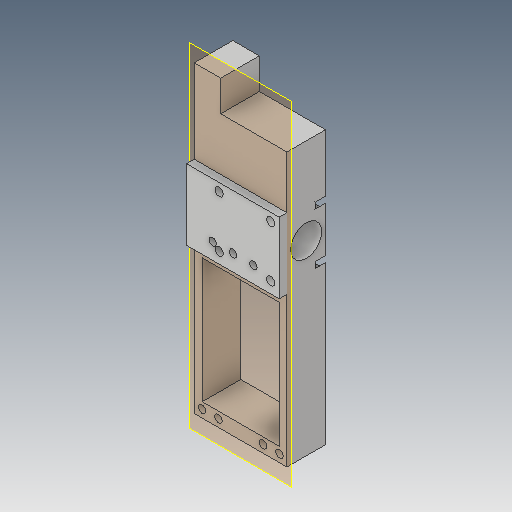
# Autodesk Inventor part: 01_Slide_camera_x_rail
Saved by Autodesk Inventor 2019.4 (Build 234330000, 330)
## iProperties
Created: 2021-01-10
Part Number: 01_Slide_camera_x_rail
Material: Generic
Document SubType Name: Modeling
Designer: diederichbenedict
Density: 1 g/cm^3
Appearance: Default
Author: diederichbenedict
Autodesk Inventor part; units mm, degrees
ref_plane "YZ Plane" through (0, 0, 0) normal (1, 0, 0) x (0, 1, 0)
ref_plane "XZ Plane" through (0, 0, 0) normal (0, 1, 0) x (-1, 0, 0)
ref_plane "Work Plane1" through (0, 0, 0) normal (0, 0, 1) x (1, 0, 0)
sketch "Sketch1" plane through (0, 0, 0) normal (0, 0, 1) x (1, 0, 0)
  line L0 (-14.0647, -9.1525) -> (-14.0647, 39.2801) projected
  line L1 (15.9353, 39.2801) -> (-14.0647, 39.2801) projected
  line L2 (15.9353, 39.2801) -> (15.9353, -9.1525) projected
  line L3 (15.9353, -9.1525) -> (-14.0647, -9.1525) projected
  circle A0 centre (13.8475, 49.7489) radius 1.45 projected
  circle A1 centre (-6.9768, 49.7489) radius 1.45 projected
  circle A2 centre (15.9823, -11.6603) radius 1.45 projected
  circle A3 centre (9.593, -11.6603) radius 1.45 projected
  circle A4 centre (-7.7223, -11.6603) radius 1.45 projected
  circle A5 centre (-14.1116, -11.6603) radius 1.45 projected
  circle A6 centre (8.8475, 49.7489) radius 1.45 projected
  circle A7 centre (-11.9768, 49.7489) radius 1.45 projected
  circle A8 centre (0.9375, 49.7489) radius 1.45 projected
  line L4 (-17.1585, 69.3865) -> (-2.1585, 69.3865) projected
  line L5 (-2.1585, 69.3865) -> (-2.1585, 62.7008) projected
  line L6 (-2.1585, 62.7008) -> (-2.1585, 59.9787) projected
  line L7 (-2.1585, 59.9787) -> (-2.1585, 53.293) projected
  line L8 (-2.1585, 53.293) -> (-17.1585, 53.293) projected
  line L9 (-17.1585, 53.293) -> (-17.1585, -14.6603) projected
  line L10 (-17.1585, -14.6603) -> (18.8415, -14.6603) projected
  line L11 (18.8415, -14.6603) -> (18.8415, 91.3397) projected
  line L12 (-6.8647, 91.3397) -> (18.8415, 91.3397) projected
  line L13 (-6.8647, 103.3397) -> (-6.8647, 91.3397) projected
  line L14 (-17.1585, 69.3865) -> (-17.1585, 103.3397) projected
  line L15 (-17.1585, 69.3865) -> (-17.1585, 53.293)
  line L16 (-17.1585, 103.3397) -> (-6.8647, 103.3397) projected
  point P0 (0, 0)
  constraints: 2 end point, 1 vertical
ref_plane "Work Plane2" through (-17.2444, -14.6603, -15) normal (0, 0, 1) x (1, 0, 0)
extrude "Extrusion1" add sketch "Sketch1" against normal up to surface (15 mm away) contours A0 | A7 | L14 L16 L13 L12 L11 L10 L9 L8 L7 L6 L5 L4 | L4 L5 L6 L7 L8 L15
sketch "Sketch2" plane through (-17.1585, -14.6603, 0) normal (-1, 0, 0) x (0, 0, 1)
  line L0 (-15, 0) -> (-15, 118) projected
  line L1 (0, 0) -> (-15, 0) projected
  line L2 (0, 118) -> (0, 0) projected
  line L3 (0, 118) -> (-15, 118) projected
  line L4 (9.1746, 66.4404) -> (8.5, 66.4404) projected
  line L5 (8.5, 78.4403) -> (9.1746, 78.4403) projected
  circle A0 centre (-7.5, 72.4403) radius 6.0376
  point P0 (0, 14.6603)
  dimension "d2" = 6
  dimension "d3" = 7.5
  constraints: 1 centre point
  measures "d2" distance from line of A0.centre L5
  measures "d3" distance from line of A0.centre L2
extrude "Extrusion2" cut sketch "Sketch2" against normal through all contours A0
sketch "Sketch3" plane through (-17.1585, -14.6603, 0) normal (-1, 0, 0) x (0, 0, 1)
  circle A0 centre (-7.5, 64.4403) radius 1.625 projected
  circle A1 centre (-7.5, 72.4403) radius 6.0376 projected
  line L0 (-15, 0) -> (-15, 118) projected
  line L1 (0, 0) -> (-15, 0) projected
  line L2 (0, 118) -> (0, 0) projected
  line L3 (0, 118) -> (-15, 118) projected
  circle A2 centre (-7.5, 80.4403) radius 1.625 projected
  circle A3 centre (-7.5, 80.4403) radius 1.45
  circle A4 centre (-7.5, 64.4403) radius 1.45
  point P0 (0, 14.6603)
  dimension "d6" = 2.9
  dimension "d7" = 2.9
  constraints: 2 centre point, 2 coincident
  measures "d6" diameter of A3
  measures "d7" diameter of A4
extrude "Extrusion3" cut sketch "Sketch3" against normal blind 20 contours A3 | A4
sketch "Sketch4" plane through (18.8415, -14.6603, -15) normal (0, 0, -1) x (-1, 0, 0)
  circle A0 centre (3.3, 62.4404) radius 1.25 projected
  circle A1 centre (3.3, 82.4404) radius 1.25 projected
  circle A2 centre (23.3, 82.4404) radius 1.5 projected
  circle A3 centre (23.3, 62.4404) radius 1.75 projected
  point P0 (18.8415, 14.6603)
hole "Hole1" at (-4.4585, 47.7801, -15) at (-4.4585, 67.7801, -15) at (15.5415, 67.7801, -15) at (15.5415, 47.7801, -15) direction (0, 0, 1) diameter 3.2 end through all counterbore diameter 7 counterbore depth 4
sketch "Sketch5" plane through (0, 0, 0) normal (0, 0, 1) x (1, 0, 0)
  circle A0 centre (15.5415, 47.7801) radius 1.6 projected
  circle A1 centre (15.5415, 67.7801) radius 1.6 projected
  circle A2 centre (-4.4585, 47.7801) radius 1.6 projected
  circle A3 centre (-4.4585, 67.7801) radius 1.6 projected
  line L0 (15.9353, -9.1525) -> (-14.0647, -9.1525) projected
  line L1 (-14.0647, -9.1525) -> (-14.0647, 39.2801) projected
  line L2 (-14.0647, 39.2801) -> (15.9353, 39.2801) projected
  line L3 (15.9353, 39.2801) -> (15.9353, -9.1525) projected
  circle A4 centre (0.9375, 49.7489) radius 1.45 projected
  circle A5 centre (8.8475, 49.7489) radius 1.45 projected
  circle A6 centre (-14.1116, -11.6603) radius 1.45 projected
  circle A7 centre (-7.7223, -11.6603) radius 1.45 projected
  circle A8 centre (9.593, -11.6603) radius 1.45 projected
  circle A9 centre (15.9823, -11.6603) radius 1.45 projected
  circle A10 centre (-6.9768, 49.7489) radius 1.45 projected
  line L4 (-17.1585, 103.3397) -> (-17.1585, -14.6603) projected
  line L5 (-17.1585, -14.6603) -> (18.8415, -14.6603) projected
  line L6 (18.8415, -14.6603) -> (18.8415, 91.3397) projected
  line L7 (18.8415, 91.3397) -> (-6.8647, 91.3397) projected
  line L8 (-6.8647, 91.3397) -> (-6.8647, 103.3397) projected
  line L9 (-6.8647, 103.3397) -> (-17.1585, 103.3397) projected
  line L10 (-17.1585, 70.9125) -> (18.8415, 70.9125)
  line L11 (18.8415, 70.9125) -> (18.8415, 43.4454)
  line L12 (18.8415, 43.4454) -> (-17.1585, 43.4454)
  line L13 (-17.1585, 43.4454) -> (-17.1585, 70.9125)
  point P0 (0, 0)
  constraints: 8 end point, 2 parallel, 2 point on line, 1 horizontal, 1 perpendicular
extrude "Extrusion4" add sketch "Sketch5" along normal blind 3 contours L10 L6 L12 L4
body "Solid1"
